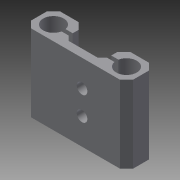
# Autodesk Inventor part: ChimeraXCarriageLowTest
Saved by Autodesk Inventor 2015 SP1 (Build 190203100, 203)
## iProperties
Created: 2015-03-09
Part Number: ChimeraXCarriageLowTest
Material: Generic
Document SubType Name: Modeling
Designer: Jack
Density: 1 g/cm^3
Appearance: Default
Author: Jack
Autodesk Inventor part; units mm, degrees
ref_plane "YZ Plane" through (0, 0, 0) normal (1, 0, 0) x (0, 1, 0)
ref_plane "XZ Plane" through (0, 0, 0) normal (0, 1, 0) x (-1, 0, 0)
ref_plane "XY Plane" through (0, 0, 0) normal (0, 0, 1) x (1, 0, 0)
sketch "Sketch1" plane through (0, 0, 0) normal (0, 0, 1) x (1, 0, 0)
  arc A0 (7.6035, 1.5) -> (7.6035, -1.5) centre (0, 0) ccw
  arc A1 (47.3965, -1.5) -> (47.3965, 1.5) centre (55, 0) ccw
  line L0 (-11, -11) -> (66, -11)
  line L1 (66, -11) -> (66, 11)
  line L2 (66, 11) -> (42, 11)
  line L3 (42, 11) -> (42, 1.5)
  line L4 (42, 1.5) -> (47.3965, 1.5)
  line L5 (13, 11) -> (-11, 11)
  line L6 (-11, 11) -> (-11, -11)
  line L7 (13, 11) -> (13, 1.5)
  line L8 (13, 1.5) -> (7.6035, 1.5)
  line L9 (7.6035, -1.5) -> (13, -1.5)
  line L10 (13, -1.5) -> (13, -5)
  line L11 (13, -5) -> (42, -5)
  line L12 (42, -5) -> (42, -1.5)
  line L13 (42, -1.5) -> (47.3965, -1.5)
  dimension "d0" = 15.5
  dimension "d1" = 55
  dimension "d2" = 11
  dimension "d3" = 11
  dimension "d4" = 11
  dimension "d7" = 1.5
  dimension "d8" = 1.5
  dimension "d9" = 13
  dimension "d10" = 13
  dimension "d11" = 6
  constraints: 28 end point, 9 perpendicular, 4 point on circle, 4 point on line, 2 centre point, 2 horizontal, 2 horizontal alignment, 2 vertical alignment, 1 coincident, 1 collinear, 1 equal radius, 1 vertical
  measures "d0" diameter of A0
  measures "d1" distance of point (0, 0) A1.centre
  measures "d2" distance from line of point (0, 0) L0
  measures "d3" distance from line of point (0, 0) L6
  measures "d4" distance from line of L5 point (0, 0)
  measures "d7" distance from line of point (0, 0) L9
  measures "d8" distance from line of point (0, 0) L8
  measures "d9" distance from line of A1.centre L12
  measures "d10" distance from line of point (0, 0) L10
  measures "d11" distance between parallel lines of L0 L11
extrude "Extrusion1" add sketch "Sketch1" along normal blind 58
chamfer "Chamfer1" distance 5 angle 45 6 edges at (-11, 11, 29) (-11, -11, 29) (66, 11, 29) (66, -11, 29) (42, 11, 29) (13, 11, 29)
chamfer "Chamfer2" distance 3.5 angle 45 2 edges at (42, -5, 29) (13, -5, 29)
sketch "Sketch2" plane through (16.5, -5, 0) normal (0, 1, 0) x (1, 0, 0)
  line L0 (22, 0) -> (22, -58) projected
  line L1 (22, 0) -> (0, 0) projected
  circle A0 centre (16, -20) radius 4
  circle A1 centre (16, -38) radius 4
  point P0 (-16.5, 0)
  dimension "d20" = 8
  dimension "d21" = 6
  dimension "d22" = 20
  dimension "d23" = 18
  constraints: 2 centre point, 1 equal radius, 1 vertical alignment
  measures "d20" diameter of A0
  measures "d21" distance from line of L0 A0.centre
  measures "d22" distance from line of L1 A0.centre
  measures "d23" distance of A0.centre A1.centre
extrude "Extrusion2" cut sketch "Sketch2" against normal up to next
body "Solid1"
